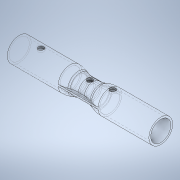
# Autodesk Inventor part: Venturi Valve
Saved by Autodesk Inventor 2021 (Build 250183000, 183)
## iProperties
Created: 2020-04-18
Part Number: Venturi Valve
Material: Generic
Document SubType Name: Modeling
Designer: James
Density: 1 g/cm^3
Appearance: Semi-Polished
Author: James
Autodesk Inventor part; units mm, degrees
ref_plane "YZ Plane" through (0, 0, 0) normal (1, 0, 0) x (0, 1, 0)
ref_plane "XZ Plane" through (0, 0, 0) normal (0, 1, 0) x (-1, 0, 0)
ref_plane "XY Plane" through (0, 0, 0) normal (0, 0, 1) x (1, 0, 0)
sketch "Sketch1" plane through (0, 0, 0) normal (0, 0, 1) x (1, 0, 0)
  line L0 (0, 0) -> (70, 0)
  line L1 (23.4899, 8.9035) -> (21.5101, 9.5965)
  line L2 (46.5101, 8.9035) -> (48.4899, 9.5965)
  arc A0 (21.5101, 9.5965) -> (13.2514, 11) centre (13.2514, -14) ccw
  arc A1 (23.4899, 8.9035) -> (31.7486, 7.5) centre (31.7486, 32.5) ccw
  arc A2 (38.2514, 7.5) -> (46.5101, 8.9035) centre (38.2514, 32.5) ccw
  arc A3 (56.7486, 11) -> (48.4899, 9.5965) centre (56.7486, -14) ccw
  arc A4 (22.1708, 11.4842) -> (13.2514, 13) centre (13.2514, -14) ccw
  line L3 (22.1708, 11.4842) -> (24.1506, 10.7913)
  arc A5 (24.1506, 10.7913) -> (31.7486, 9.5) centre (31.7486, 32.5) ccw
  arc A6 (38.2514, 9.5) -> (45.8494, 10.7913) centre (38.2514, 32.5) ccw
  line L4 (45.8494, 10.7913) -> (47.8292, 11.4842)
  arc A7 (56.7486, 13) -> (47.8292, 11.4842) centre (56.7486, -14) ccw
  line L5 (31.7486, 9.5) -> (38.2514, 9.5)
  line L6 (31.7486, 7.5) -> (38.2514, 7.5)
  line L7 (-42.25, 13) -> (-42.25, 11)
  line L8 (112.25, 13) -> (112.25, 11)
  line L9 (56.7486, 13) -> (112.25, 13)
  line L10 (56.7486, 11) -> (112.25, 11)
  line L11 (13.2514, 13) -> (-42.25, 13)
  line L12 (13.2514, 11) -> (-42.25, 11)
  point P0 (17.5, 11)
  point P1 (52.5, 11)
  point P2 (42.5, 7.5)
  point P3 (27.5, 7.5)
  dimension "d8" = 25
  dimension "d43" = 154.5
  constraints: 26 end point, 16 point on circle, 8 centre point, 5 horizontal, 4 point on line, 2 vertical
  measures "d8" radius of A0
  measures "d43" distance from line of L8.start L7
revolve "Revolution1" add sketch "Sketch1" angle 360 about axis through (0, 0, 0) along (1, 0, 0)
sketch "Sketch3" plane through (0, 0, 0) normal (0, 1, 0) x (-1, 0, 0)
  circle A0 centre (-35, 0) radius 3
  line L0 (-70, 11) -> (-70, -11) projected
  line L1 (-56.7486, 11) -> (-56.7486, -11) projected
  line L2 (-70, 0) -> (-60, 0)
  circle A1 centre (-60, 0) radius 3
  line L3 (-13.2514, 11) -> (-13.2514, -11) projected
  circle A2 centre (18.2486, 0) radius 3
  dimension "d12" = 6
  dimension "d13" = 10
  dimension "d14" = 6
  dimension "d51" = 6
  constraints: 3 centre point, 2 end point, 1 coincident, 1 horizontal, 1 midpoint
  measures "d12" diameter of A0
  measures "d13" distance of L2.start L2.end
  measures "d14" diameter of A1
  measures "d51" diameter of A2
extrude "Extrusion1" cut sketch "Sketch3" along normal blind 20
sketch "Sketch4" plane through (0, 0, 0) normal (0, 1, 0) x (-1, 0, 0)
  line L0 (-56.7486, -13) -> (-13.2514, -13)
  arc A0 (-56.7486, -12) -> (-48.1595, -10.5403) centre (-56.7486, 14) ccw
  line L1 (-48.1595, -10.5403) -> (-46.1798, -9.8474)
  arc A1 (-38.2514, -8.5) -> (-46.1798, -9.8474) centre (-38.2514, -32.5) ccw
  line L2 (-31.7486, -8.5) -> (-38.2514, -8.5)
  arc A2 (-23.8202, -9.8474) -> (-31.7486, -8.5) centre (-31.7486, -32.5) ccw
  line L3 (-23.8202, -9.8474) -> (-21.8405, -10.5403)
  arc A3 (-21.8405, -10.5403) -> (-13.2514, -12) centre (-13.2514, 14) ccw
  line L4 (-56.7486, -13) -> (-56.7486, -12)
  line L5 (-13.2514, -12) -> (-13.2514, -13)
  point P0 (0, 0)
  point P1 (-22.1708, -11.4842)
  point P2 (-38.2514, -9.5)
  point P3 (-45.8494, -10.7913)
  point P4 (-47.8292, -11.4842)
  point P5 (-38.2514, -8.5)
  point P6 (-48.1595, -10.5403)
  constraints: 12 end point, 8 point on circle, 4 centre point
extrude "Extrusion3" add sketch "Sketch4" along normal mid plane 2
mirror "Mirror1" about plane through (0, 0, 0) normal (0, 0, 1) of "Extrusion3"
sketch "Sketch6" plane through (-42.25, 0, 0) normal (-1, 0, 0) x (0, 0, 1)
  line L0 (13, 1) -> (13, 0) projected
  circle A0 centre (0, 0) radius 13
  circle A1 centre (0, 0) radius 15
  dimension "d46" = 30
  constraints: 2 coincident, 1 centre point, 1 horizontal alignment, 2 other
  measures "d46" diameter of A1
extrude "Extrusion6" cut sketch "Sketch6" against normal up to surface (154.5 mm away)
body "Solid1"
